Autodesk Fusion 360 part; units mm, degrees
(part 13 of 13)
  line L10724 (117.495, -110.761) -> (117.499, -110.754)
  line L10725 (117.587, -112.069) -> (117.579, -112.039)
  line L10726 (118.525, -112.429) -> (118.495, -112.435)
  line L10727 (119.85, -112.485) -> (119.85, -112.335)
  line L10728 (118.466, -112.444) -> (117.983, -112.444)
  line L10729 (117.947, -112.439) -> (117.922, -112.422)
  line L10730 (115.743, -113.759) -> (122.686, -113.759)
  line L10731 (117.956, -112.441) -> (117.954, -112.44)
  line L10732 (122.467, -112.483) -> (122.453, -112.466)
  line L10733 (123.116, -113.101) -> (123.113, -113.101)
  line L10734 (123.08, -113.084) -> (123.051, -113.068)
  line L10735 (117.506, -110.75) -> (117.513, -110.748)
  line L10736 (123.051, -113.068) -> (122.467, -112.483)
  line L10737 (117.513, -111.938) -> (117.506, -111.937)
  line L10738 (117.579, -112.039) -> (117.579, -111.938)
  line L10739 (117.513, -110.748) -> (117.873, -110.748)
  line L10740 (118.55, -112.41) -> (118.536, -112.421)
  line L10741 (122.445, -112.455) -> (122.442, -112.439)
  line L10742 (123.349, -113.096) -> (123.144, -113.104)
  line L10743 (117.881, -110.75) -> (117.887, -110.754)
  line L10744 (121.93, -112.439) -> (121.834, -112.42)
  line L10745 (118.495, -112.435) -> (118.466, -112.444)
  line L10746 (123.111, -113.101) -> (123.109, -113.1)
  line L10747 (122.453, -112.466) -> (122.45, -112.463)
  line L10748 (117.873, -110.748) -> (117.881, -110.75)
  line L10749 (120.85, -111.86) -> (120.85, -112.485)
  line L10750 (119.85, -112.335) -> (119.55, -112.335)
  line L10751 (117.887, -110.754) -> (117.892, -110.761)
  line L10752 (117.495, -111.926) -> (117.493, -111.918)
  line L10753 (117.493, -111.918) -> (117.493, -110.768)
  line L10754 (118.53, -112.425) -> (118.525, -112.429)
  line L10755 (117.602, -112.11) -> (117.598, -112.107)
  line L10756 (117.954, -112.44) -> (117.947, -112.439)
  line L10757 (117.895, -112.407) -> (117.615, -112.128)
  line L10758 (121.68, -111.86) -> (120.85, -111.86)
  line L10759 (122.686, -113.759) -> (123.349, -113.096)
  line L10760 (117.579, -111.938) -> (117.513, -111.938)
  line L10761 (117.615, -112.128) -> (117.602, -112.11)
  line L10762 (121.699, -112.284) -> (121.68, -112.189)
  line L10763 (122.449, -112.46) -> (122.445, -112.455)
  line L10764 (123.144, -113.104) -> (123.116, -113.101)
  line L10765 (117.499, -111.932) -> (117.495, -111.926)
  line L10766 (117.983, -112.444) -> (117.961, -112.441)
  line L10767 (117.598, -112.104) -> (117.594, -112.099)
  line L10768 (120.85, -112.485) -> (119.85, -112.485)
  line L10769 (117.506, -111.937) -> (117.499, -111.932)
  line L10770 (117.493, -110.768) -> (117.495, -110.761)
  line L10771 (117.598, -112.107) -> (117.598, -112.104)
  line L10772 (123.43, -112.189) -> (123.411, -112.284)
  line L10773 (125.714, -111.333) -> (125.795, -111.387)
  line L10774 (118.55, -110.985) -> (119.55, -110.985)
  line L10775 (117.829, -111.988) -> (118.035, -112.194)
  line L10776 (123.357, -111.387) -> (123.411, -111.468)
  line L10777 (120.85, -110.985) -> (120.85, -111.61)
  line L10778 (123.276, -112.42) -> (123.18, -112.439)
  line L10779 (120.85, -111.61) -> (121.68, -111.61)
  line L10780 (124.118, -112.189) -> (124.118, -111.564)
  line L10781 (123.43, -111.564) -> (123.43, -112.189)
  line L10782 (117.499, -110.754) -> (117.506, -110.75)
  line L10783 (118.414, -112.194) -> (118.55, -112.058)
  line L10784 (121.699, -111.468) -> (121.753, -111.387)
  line L10785 (124.118, -111.564) -> (124.137, -111.468)
  line L10786 (123.394, -112.83) -> (123.451, -112.719)
  line L10787 (121.68, -111.564) -> (121.699, -111.468)
  line L10788 (123.276, -111.333) -> (123.357, -111.387)
  line L10789 (117.881, -111.937) -> (117.873, -111.938)
  line L10790 (121.834, -111.333) -> (121.93, -111.314)
  line L10791 (117.892, -110.761) -> (117.893, -110.768)
  line L10792 (117.961, -112.441) -> (117.956, -112.441)
  line L10793 (117.922, -112.422) -> (117.895, -112.407)
  line L10794 (118.55, -112.058) -> (118.55, -110.985)
  line L10795 (117.873, -111.938) -> (117.829, -111.938)
  line L10796 (119.85, -110.985) -> (120.85, -110.985)
  line L10797 (119.85, -111.135) -> (119.85, -110.985)
  line L10798 (123.18, -111.314) -> (123.276, -111.333)
  line L10799 (124.192, -112.366) -> (124.137, -112.284)
  line L10800 (117.887, -111.932) -> (117.881, -111.937)
  line L10801 (119.55, -111.135) -> (119.85, -111.135)
  line L10802 (117.594, -112.099) -> (117.587, -112.069)
  line L10803 (117.829, -111.938) -> (117.829, -111.988)
  line L10804 (124.368, -112.439) -> (124.273, -112.42)
  line L10805 (117.892, -111.926) -> (117.887, -111.932)
  line L10806 (118.035, -112.194) -> (118.414, -112.194)
  line L10807 (124.273, -112.42) -> (124.192, -112.366)
  line L10808 (124.009, -112.63) -> (124.098, -112.719)
  line L10809 (117.893, -111.918) -> (117.892, -111.926)
  line L10810 (121.93, -111.314) -> (123.18, -111.314)
  line L10811 (119.55, -110.985) -> (119.55, -111.135)
  line L10812 (124.137, -111.468) -> (124.192, -111.387)
  line L10813 (123.411, -112.284) -> (123.357, -112.366)
  line L10814 (121.753, -111.387) -> (121.834, -111.333)
  line L10815 (123.411, -111.468) -> (123.43, -111.564)
  line L10816 (117.893, -110.768) -> (117.893, -111.918)
  line L10817 (121.68, -111.61) -> (121.68, -111.564)
  line L10818 (124.192, -111.387) -> (124.273, -111.333)
  line L10819 (124.273, -111.333) -> (124.368, -111.314)
  line L10820 (127.954, -111.059) -> (127.96, -111.049)
  line L10821 (123.392, -112.844) -> (123.394, -112.83)
  line L10822 (124.368, -111.314) -> (125.618, -111.314)
  line L10823 (125.618, -111.314) -> (125.714, -111.333)
  line L10824 (124.158, -113.055) -> (124.289, -113.186)
  line L10825 (128.564, -110.437) -> (128.575, -110.434)
  line L10826 (127.96, -111.049) -> (127.963, -111.038)
  line L10827 (128.538, -110.458) -> (128.564, -110.437)
  line L10828 (123.898, -112.573) -> (124.009, -112.63)
  line L10829 (125.849, -112.284) -> (125.795, -112.366)
  line L10830 (124.098, -112.719) -> (124.111, -112.745)
  line L10831 (124.771, -112.439) -> (124.159, -113.051)
  line L10832 (124.159, -113.051) -> (124.158, -113.055)
  line L10833 (128.651, -110.417) -> (136.068, -110.417)
  line L10834 (128.585, -110.428) -> (128.618, -110.424)
  line L10835 (119.55, -111.535) -> (119.55, -111.935)
  line L10836 (123.18, -112.439) -> (122.776, -112.439)
  line L10837 (123.451, -112.719) -> (123.539, -112.63)
  line L10838 (125.618, -112.439) -> (124.771, -112.439)
  line L10839 (127.273, -113.186) -> (127.943, -112.515)
  line L10840 (125.849, -111.468) -> (125.868, -111.564)
  line L10841 (124.137, -112.284) -> (124.118, -112.189)
  line L10842 (125.868, -111.564) -> (125.868, -112.189)
  line L10843 (125.868, -112.189) -> (125.849, -112.284)
  line L10844 (125.795, -111.387) -> (125.849, -111.468)
  line L10845 (123.357, -112.366) -> (123.276, -112.42)
  line L10846 (122.776, -112.439) -> (123.189, -112.852)
  line L10847 (119.85, -111.935) -> (119.85, -111.535)
  line L10848 (128.51, -110.475) -> (128.538, -110.458)
  line L10849 (136.068, -110.417) -> (136.101, -110.424)
  line L10850 (124.417, -112.439) -> (124.368, -112.439)
  line L10851 (119.85, -111.535) -> (119.55, -111.535)
  line L10852 (123.651, -112.573) -> (123.774, -112.554)
  line L10853 (123.539, -112.63) -> (123.651, -112.573)
  line L10854 (124.111, -112.745) -> (124.417, -112.439)
  line L10855 (123.774, -112.554) -> (123.898, -112.573)
  line L10856 (125.795, -112.366) -> (125.714, -112.42)
  line L10857 (128.575, -110.434) -> (128.585, -110.428)
  line L10858 (124.289, -113.186) -> (127.273, -113.186)
  line L10859 (119.55, -111.935) -> (119.85, -111.935)
  line L10860 (123.189, -112.852) -> (123.392, -112.844)
  line L10861 (128.618, -110.424) -> (128.651, -110.417)
  line L10862 (144.49, -111.398) -> (144.544, -111.479)
  line L10863 (144.544, -111.479) -> (144.563, -111.574)
  line L10864 (127.943, -111.125) -> (127.95, -111.092)
  line L10865 (125.714, -112.42) -> (125.618, -112.439)
  line L10866 (144.408, -111.343) -> (144.49, -111.398)
  line L10867 (128.002, -110.984) -> (128.51, -110.475)
  line L10868 (144.479, -113.126) -> (144.474, -113.127)
  line L10869 (145.401, -112.376) -> (145.346, -112.295)
  line L10870 (144.122, -112.449) -> (144.552, -112.88)
  line L10871 (145.465, -112.83) -> (145.485, -112.954)
  line L10872 (144.552, -112.88) -> (144.697, -112.88)
  line L10873 (145.465, -113.077) -> (145.408, -113.189)
  line L10874 (127.984, -111.012) -> (128.002, -110.984)
  line L10875 (142.832, -111.479) -> (142.886, -111.398)
  line L10876 (144.961, -113.334) -> (144.85, -113.277)
  line L10877 (145.261, -112.6) -> (145.452, -112.41)
  line L10878 (144.313, -112.449) -> (144.122, -112.449)
  line L10879 (144.85, -112.63) -> (144.961, -112.573)
  line L10880 (145.327, -111.574) -> (145.346, -111.479)
  line L10881 (144.408, -112.43) -> (144.313, -112.449)
  line L10882 (144.761, -112.719) -> (144.85, -112.63)
  line L10883 (144.961, -112.573) -> (145.085, -112.554)
  line L10884 (145.346, -112.295) -> (145.327, -112.199)
  line L10885 (146.827, -111.324) -> (146.923, -111.343)
  line L10886 (127.963, -111.038) -> (127.984, -111.012)
  line L10887 (144.49, -112.376) -> (144.408, -112.43)
  line L10888 (144.544, -112.295) -> (144.49, -112.376)
  line L10889 (145.452, -112.41) -> (145.401, -112.376)
  line L10890 (145.346, -111.479) -> (145.401, -111.398)
  line L10891 (147.077, -112.199) -> (147.058, -112.295)
  line L10892 (147.077, -111.574) -> (147.077, -112.199)
  line L10893 (144.704, -112.83) -> (144.761, -112.719)
  line L10894 (144.474, -113.127) -> (144.471, -113.125)
  line L10895 (145.327, -112.199) -> (145.327, -111.574)
  line L10896 (145.208, -112.573) -> (145.261, -112.6)
  line L10897 (144.412, -113.093) -> (143.769, -112.449)
  line L10898 (145.32, -113.277) -> (145.208, -113.334)
  line L10899 (145.766, -112.449) -> (145.438, -112.777)
  line L10900 (146.923, -111.343) -> (147.004, -111.398)
  line L10901 (144.563, -111.574) -> (144.563, -112.199)
  line L10902 (127.943, -112.515) -> (127.943, -111.125)
  line L10903 (144.563, -112.199) -> (144.544, -112.295)
  line L10904 (145.085, -112.554) -> (145.208, -112.573)
  line L10905 (145.401, -111.398) -> (145.482, -111.343)
  line L10906 (144.697, -112.88) -> (144.704, -112.83)
  line L10907 (147.058, -112.295) -> (147.004, -112.376)
  line L10908 (145.577, -111.324) -> (146.827, -111.324)
  line L10909 (147.058, -111.479) -> (147.077, -111.574)
  line L10910 (127.95, -111.092) -> (127.954, -111.059)
  line L10911 (147.004, -111.398) -> (147.058, -111.479)
  line L10912 (145.085, -113.354) -> (144.961, -113.334)
  line L10913 (144.85, -113.277) -> (144.761, -113.189)
  line L10914 (145.482, -111.343) -> (145.577, -111.324)
  line L10915 (145.408, -113.189) -> (145.32, -113.277)
  line L10916 (107.414, -117.855) -> (107.675, -118.116)
  line L10917 (107.703, -118.175) -> (107.712, -118.204)
  line L10918 (107.462, -118.256) -> (107.238, -118.032)
  line L10919 (106.661, -117.678) -> (106.681, -117.555)
  line L10920 (107.499, -122.915) -> (107.485, -122.898)
  line L10921 (107.862, -123.278) -> (107.862, -123.278)
  line L10922 (107.481, -122.892) -> (107.477, -122.887)
  line L10923 (146.78, -96.8204) -> (146.765, -96.8969)
  line L10924 (106.737, -117.913) -> (106.681, -117.802)
  line L10925 (145.98, -96.2704) -> (145.995, -96.1939)
  line L10926 (108.038, -123.102) -> (108.038, -123.102)
  line L10927 (106.737, -117.443) -> (106.826, -117.355)
  line L10928 (107.712, -118.204) -> (107.712, -122.775)
  line L10929 (108.967, -124.03) -> (141.756, -124.03)
  line L10930 (107.441, -117.802) -> (107.414, -117.855)
  line L10931 (107.471, -122.857) -> (107.462, -122.827)
  line L10932 (107.477, -122.887) -> (107.471, -122.857)
  line L10933 (146.722, -96.129) -> (146.765, -96.1939)
  line L10934 (107.238, -118.032) -> (107.185, -118.059)
  line L10935 (107.441, -117.555) -> (107.461, -117.678)
  line L10936 (108.886, -124.276) -> (108.88, -124.275)
  line L10937 (106.681, -117.555) -> (106.737, -117.443)
  line L10938 (146.18, -96.0704) -> (146.58, -96.0704)
  line L10939 (107.385, -117.443) -> (107.441, -117.555)
  line L10940 (107.461, -117.678) -> (107.441, -117.802)
  line L10941 (107.712, -122.775) -> (108.038, -123.102)
  line L10942 (107.296, -117.355) -> (107.385, -117.443)
  line L10943 (108.827, -124.244) -> (107.862, -123.278)
  line L10944 (106.681, -117.802) -> (106.661, -117.678)
  line L10945 (106.937, -117.298) -> (107.061, -117.278)
  line L10946 (145.995, -96.1939) -> (146.039, -96.129)
  line L10947 (108.889, -124.277) -> (108.886, -124.276)
  line L10948 (146.039, -96.129) -> (146.104, -96.0856)
  line L10949 (106.826, -117.355) -> (106.937, -117.298)
  line L10950 (107.697, -118.145) -> (107.703, -118.175)
  line L10951 (108.915, -124.28) -> (108.893, -124.277)
  line L10952 (107.862, -123.278) -> (107.499, -122.915)
  line L10953 (141.837, -124.272) -> (141.807, -124.28)
  line L10954 (108.88, -124.275) -> (108.854, -124.258)
sketch "Sketch2" plane through (0, 0, 0) normal (0, 0, 1) x (1, 0, 0)
  line L0 (149, -96) -> (101, -96)
  line L1 (101, -96) -> (101, -78)
  line L2 (101, -78) -> (149, -78)
  line L3 (149, -78) -> (149, -96)
  constraint horizontal L0
  constraint vertical L1
  constraint horizontal L2
  constraint vertical L3
extrude "Extrude1" add sketch "Sketch2" along normal blind 1
sketch "Sketch3" plane through (0, 0, 0) normal (0, 0, -1) x (-1, 0, 0)
  line L0 (-101, -78) -> (-149, -78)
  line L1 (-149, -78) -> (-149, -96)
  line L2 (-149, -96) -> (-101, -96)
  line L3 (-101, -96) -> (-101, -78)
  circle A0 centre (-108.7784, -82.0867) radius 0.675
  circle A1 centre (-107.4474, -84.686) radius 0.675
  circle A2 centre (-112.6298, -84.6454) radius 0.675
  circle A3 centre (-108.8729, -86.028) radius 0.675
  circle A4 centre (-107.4551, -87.3247) radius 0.675
  circle A5 centre (-111.5378, -87.2373) radius 0.675
  circle A6 centre (-112.8215, -88.5302) radius 0.675
  circle A7 centre (-111.7823, -89.8823) radius 0.675
  circle A8 centre (-108.2, -89.85) radius 0.675
  circle A9 centre (-109.8635, -92.6666) radius 0.675
  circle A10 centre (-112.05, -92.7) radius 0.675
  circle A11 centre (-114.0365, -92.6228) radius 0.675
  circle A12 centre (-117.8364, -92.898) radius 0.675
  circle A13 centre (-120.63, -92.69) radius 0.675
  circle A14 centre (-123.9456, -92.7311) radius 0.675
  circle A15 centre (-129.9244, -91.2828) radius 0.675
  circle A16 centre (-133.85, -91.1) radius 0.675
  circle A17 centre (-141.5, -92.26) radius 0.675
  circle A18 centre (-136, -83.2) radius 0.675
  circle A19 centre (-136, -86.2325) radius 0.675
  circle A20 centre (-140.7296, -81.6222) radius 0.675
  circle A21 centre (-130.6, -85.2) radius 0.675
  circle A22 centre (-129.5, -81.8) radius 0.675
  circle A23 centre (-126.6, -82.9) radius 0.675
  circle A24 centre (-124.65, -81.65) radius 0.675
  circle A25 centre (-122.1992, -81.5755) radius 0.675
  dimension "d5" = 1.35
  dimension "d6" = 1.35
  dimension "d7" = 1.35
  dimension "d8" = 1.35
  dimension "d9" = 1.35
  dimension "d10" = 1.35
  dimension "d11" = 1.35
  dimension "d12" = 1.35
  dimension "d13" = 1.35
  dimension "d14" = 1.35
  dimension "d15" = 1.35
  dimension "d16" = 1.35
  dimension "d17" = 1.35
  dimension "d18" = 1.35
  dimension "d19" = 1.35
  dimension "d20" = 1.35
  dimension "d21" = 1.35
  dimension "d22" = 1.35
  dimension "d23" = 1.35
  dimension "d24" = 1.35
  dimension "d25" = 1.35
  dimension "d26" = 1.35
  dimension "d27" = 1.35
  dimension "d28" = 1.35
  dimension "d29" = 1.35
  dimension "d30" = 1.35
  measures "d5" diameter of A0
  measures "d6" diameter of A1
  measures "d7" diameter of A3
  measures "d8" diameter of A4
  measures "d9" diameter of A2
  measures "d10" diameter of A5
  measures "d11" diameter of A6
  measures "d12" diameter of A7
  measures "d13" diameter of A8
  measures "d14" diameter of A9
  measures "d15" diameter of A10
  measures "d16" diameter of A11
  measures "d17" diameter of A12
  measures "d18" diameter of A13
  measures "d19" diameter of A14
  measures "d20" diameter of A15
  measures "d21" diameter of A21
  measures "d22" diameter of A23
  measures "d23" diameter of A24
  measures "d24" diameter of A25
  measures "d25" diameter of A22
  measures "d26" diameter of A16
  measures "d27" diameter of A19
  measures "d28" diameter of A18
  measures "d29" diameter of A20
  measures "d30" diameter of A17
sketch "Sketch4" plane through (0, 0, 0) normal (0, 0, -1) x (-1, 0, 0)
  line L0 (-101, -78) -> (-149, -78)
  line L1 (-149, -78) -> (-149, -96)
  line L2 (-149, -96) -> (-101, -96)
  line L3 (-101, -96) -> (-101, -78)
  line L4 (-101, -96) -> (-101, -78)
  line L5 (-149, -96) -> (-101, -96)
  circle A0 centre (-111.7823, -89.8823) radius 0.625
  circle A1 centre (-111.5378, -87.2373) radius 0.625
  circle A2 centre (-107.4474, -84.686) radius 0.625
  circle A3 centre (-141.5, -92.26) radius 0.625
  circle A4 centre (-107.4551, -87.3247) radius 0.625
  circle A5 centre (-108.7784, -82.0867) radius 0.625
  circle A6 centre (-112.8215, -88.5302) radius 0.625
  circle A7 centre (-109.8635, -92.6666) radius 0.625
  circle A8 centre (-122.1992, -81.5755) radius 0.625
  circle A9 centre (-112.6298, -84.6454) radius 0.625
  circle A10 centre (-108.2, -89.85) radius 0.625
  circle A11 centre (-136, -86.2325) radius 0.625
  circle A12 centre (-130.6, -85.2) radius 0.625
  circle A13 centre (-126.6, -82.9) radius 0.625
  circle A14 centre (-136, -83.2) radius 0.625
  circle A15 centre (-124.65, -81.65) radius 0.625
  circle A16 centre (-108.8729, -86.028) radius 0.625
  circle A17 centre (-133.85, -91.1) radius 0.625
  circle A18 centre (-114.0365, -92.6228) radius 0.625
  circle A19 centre (-117.8364, -92.898) radius 0.625
  circle A20 centre (-112.05, -92.7) radius 0.625
  circle A21 centre (-129.9244, -91.2828) radius 0.625
  circle A22 centre (-123.9456, -92.7311) radius 0.625
  circle A23 centre (-120.63, -92.69) radius 0.625
  circle A24 centre (-129.5, -81.8) radius 0.625
  line L6 (-149, -78) -> (-149, -96)
  circle A25 centre (-140.7296, -81.6222) radius 0.625
  line L7 (-101, -78) -> (-149, -78)
  dimension "d33" = 1.25
  dimension "d34" = 1.25
  dimension "d35" = 1.25
  dimension "d36" = 1.25
  dimension "d37" = 1.25
  dimension "d38" = 1.25
  dimension "d39" = 1.25
  dimension "d40" = 1.25
  dimension "d41" = 1.25
  dimension "d42" = 1.25
  dimension "d43" = 1.25
  dimension "d44" = 1.25
  dimension "d45" = 1.25
  dimension "d46" = 1.25
  dimension "d47" = 1.25
  dimension "d48" = 1.25
  dimension "d49" = 1.25
  dimension "d50" = 1.25
  dimension "d51" = 1.25
  dimension "d52" = 1.25
  dimension "d53" = 1.25
  dimension "d54" = 1.25
  dimension "d55" = 1.25
  dimension "d56" = 1.25
  dimension "d57" = 1.25
  dimension "d58" = 1.25
  measures "d33" diameter of A5
  measures "d34" diameter of A2
  measures "d35" diameter of A16
  measures "d36" diameter of A4
  measures "d37" diameter of A9
  measures "d38" diameter of A1
  measures "d39" diameter of A6
  measures "d40" diameter of A0
  measures "d41" diameter of A10
  measures "d42" diameter of A7
  measures "d43" diameter of A20
  measures "d44" diameter of A18
  measures "d45" diameter of A19
  measures "d46" diameter of A23
  measures "d47" diameter of A22
  measures "d48" diameter of A21
  measures "d49" diameter of A12
  measures "d50" diameter of A13
  measures "d51" diameter of A15
  measures "d52" diameter of A8
  measures "d53" diameter of A24
  measures "d54" diameter of A17
  measures "d55" diameter of A11
  measures "d56" diameter of A14
  measures "d57" diameter of A25
  measures "d58" diameter of A3
extrude "Extrude3" cut sketch "Sketch4" against normal blind 1 contours A0 | A1 | A2 | A3 | A4 | A5 | A6 | A7 | A8 | A9 | A10 | A11 | A12 | A13 | A14 | A15 | A16 | A17 | A18 | A19 | A20 | A21 | A22 | A23 | A24 | A25
sketch "Sketch5" plane through (0, 0, 0) normal (0, 0, -1) x (-1, 0, 0)
  circle A0 centre (-123.9456, -92.7311) radius 0.625
  circle A1 centre (-129.9244, -91.2828) radius 0.625
  circle A2 centre (-140.7296, -81.6222) radius 0.625
  circle A3 centre (-109.8635, -92.6666) radius 0.625
  circle A4 centre (-108.7784, -82.0867) radius 0.625
  circle A5 centre (-136, -83.2) radius 0.625
  circle A6 centre (-130.6, -85.2) radius 0.625
  circle A7 centre (-124.65, -81.65) radius 0.625
  circle A8 centre (-120.63, -92.69) radius 0.625
  circle A9 centre (-112.6298, -84.6454) radius 0.625
  circle A10 centre (-126.6, -82.9) radius 0.625
  circle A11 centre (-133.85, -91.1) radius 0.625
  circle A12 centre (-141.5, -92.26) radius 0.625
  circle A13 centre (-108.2, -89.85) radius 0.625
  circle A14 centre (-136, -86.2325) radius 0.625
  circle A15 centre (-129.5, -81.8) radius 0.625
  circle A16 centre (-122.1992, -81.5755) radius 0.625
  circle A17 centre (-117.8364, -92.898) radius 0.625
  line L0 (-101, -78) -> (-149, -78)
  line L1 (-149, -78) -> (-149, -96)
  line L2 (-149, -96) -> (-101, -96)
  line L3 (-101, -96) -> (-101, -78)
  circle A18 centre (-146, -93) radius 0.8
  circle A19 centre (-146, -80.9656) radius 0.8
  circle A20 centre (-103.4, -93) radius 0.8
  circle A21 centre (-103.4, -80.9656) radius 0.8
  circle A22 centre (-114.0365, -92.6228) radius 0.625
  circle A23 centre (-111.5378, -87.2373) radius 0.625
  circle A24 centre (-107.4474, -84.686) radius 0.625
  circle A25 centre (-112.8215, -88.5302) radius 0.625
  circle A26 centre (-112.05, -92.7) radius 0.625
  circle A27 centre (-107.4551, -87.3247) radius 0.625
  circle A28 centre (-108.8729, -86.028) radius 0.625
  circle A29 centre (-111.7823, -89.8823) radius 0.625
  dimension "d61" = 1.6
  dimension "d62" = 1.6
  dimension "d63" = 1.6
  dimension "d64" = 1.6
  dimension "d65" = 12.0344
  dimension "d66" = 3
  dimension "d67" = 3
  dimension "d120" = 42.6
  constraint vertical A20.centre A21.centre
  constraint vertical A18.centre A19.centre
  constraint horizontal A19.centre A21.centre
  constraint horizontal A18.centre A20.centre
  measures "d61" diameter of A18
  measures "d62" diameter of A19
  measures "d63" diameter of A20
  measures "d64" diameter of A21
  measures "d65" vertical distance of A18.centre A19.centre
  measures "d66" distance of L2 A18.centre
  measures "d67" distance of L1 A18.centre
  measures "d120" distance of A18.centre A20.centre
extrude "Extrude4" cut sketch "Sketch5" against normal blind 1 contours A18 | A19 | A20 | A21
extrude "Extrude5" add 1 faces at (117.7446, -87.5854, 0) along direction (0, 0, -1) blind 2.5
sketch "Sketch7" plane through (0, 0, 1) normal (0, 0, 1) x (1, 0, 0)
  line L0 (149, -78) -> (101, -78)
  line L1 (110.0613, -80.42) -> (140.0613, -80.42)
  line L2 (145.1, -83.5542) -> (145.1, -90.4251)
  line L3 (144.863, -82.792) -> (144.8869, -82.8311)
  line L4 (145.0782, -90.4018) -> (144.9206, -91.2794)
  line L5 (145.2412, -83.2117) -> (145.2415, -83.2103)
  line L6 (145.053, -83.4428) -> (145.1, -83.5542)
  line L7 (140.0273, -93.86) -> (110.0613, -93.86)
  line L8 (145.0889, -90.4512) -> (145.0782, -90.4018)
  line L9 (144.8869, -82.8311) -> (145.0095, -83.6161)
  line L10 (145.1, -90.4251) -> (145.0889, -90.4512)
  line L11 (145.0095, -83.6161) -> (145.053, -83.4428)
  arc A0 (110.0613, -80.42) -> (110.0613, -93.86) centre (110.0613, -87.14) ccw
  arc A1 (144.863, -82.792) -> (140.0613, -80.42) centre (140.0613, -86.4662) ccw
  arc A2 (140.0273, -93.86) -> (144.9206, -91.2794) centre (140.0273, -87.9303) ccw
  line L12 (101, -78) -> (149, -78)
  line L13 (149, -78) -> (149, -96)
  line L14 (149, -96) -> (101, -96)
  line L15 (101, -96) -> (101, -78)
  line L16 (149, -96) -> (149, -78)
  dimension "d73" = 6.72
  dimension "d75" = 6.0462
  dimension "d76" = 5.9297
  dimension "d77" = 5.0387
  dimension "d78" = 30
  dimension "d79" = 6.8709
  dimension "d80" = 2.42
  dimension "d81" = 3.9
  constraint horizontal L12
  constraint vertical L13
  constraint horizontal L14
  constraint vertical L15
  constraint coincident L0.end L12.start
  constraint collinear L13 L16
  constraint tangent L1 A0
  constraint tangent L1 A1
  constraint tangent L7 A0
  constraint tangent L7 A2
  constraint parallel L1 L7
  measures "d73" radius of A0
  measures "d75" radius of A1
  measures "d76" radius of A2
  measures "d77" distance of L2 A1.centre
  measures "d78" distance of L1.end L1.start
  measures "d79" distance of L2.start L2.end
  measures "d80" distance of L1 L12
  measures "d81" distance of L2 L13
extrude "Extrude6" add sketch "Sketch7" along normal blind 3
sketch "Sketch8" plane through (0, 0, -2.5) normal (0, 0, -1) x (-1, 0, 0)
  circle A0 centre (-146, -93) radius 0.8
  circle A1 centre (-146, -80.9656) radius 0.8
  circle A2 centre (-103.4, -93) radius 0.8
  circle A3 centre (-103.4, -80.9656) radius 0.8
  circle A4 centre (-123.9456, -92.7311) radius 0.625
  circle A5 centre (-129.9244, -91.2828) radius 0.625
  circle A6 centre (-140.7296, -81.6222) radius 0.625
  circle A7 centre (-109.8635, -92.6666) radius 0.625
  circle A8 centre (-108.7784, -82.0867) radius 0.625
  circle A9 centre (-136, -83.2) radius 0.625
  circle A10 centre (-130.6, -85.2) radius 0.625
  circle A11 centre (-124.65, -81.65) radius 0.625
  circle A12 centre (-120.63, -92.69) radius 0.625
  circle A13 centre (-112.6298, -84.6454) radius 0.625
  circle A14 centre (-126.6, -82.9) radius 0.625
  circle A15 centre (-133.85, -91.1) radius 0.625
  circle A16 centre (-141.5, -92.26) radius 0.625
  circle A17 centre (-108.2, -89.85) radius 0.625
  circle A18 centre (-136, -86.2325) radius 0.625
  circle A19 centre (-129.5, -81.8) radius 0.625
  circle A20 centre (-122.1992, -81.5755) radius 0.625
  circle A21 centre (-117.8364, -92.898) radius 0.625
  line L0 (-101, -78) -> (-149, -78)
  line L1 (-149, -78) -> (-149, -96)
  line L2 (-149, -96) -> (-101, -96)
  line L3 (-101, -96) -> (-101, -78)
  circle A22 centre (-103.4, -93) radius 0.8
  circle A23 centre (-146, -93) radius 0.8
  circle A24 centre (-146, -80.9656) radius 0.8
  circle A25 centre (-103.4, -80.9656) radius 0.8
  circle A26 centre (-114.0365, -92.6228) radius 0.625
  circle A27 centre (-111.5378, -87.2373) radius 0.625
  circle A28 centre (-107.4474, -84.686) radius 0.625
  circle A29 centre (-112.8215, -88.5302) radius 0.625
  circle A30 centre (-112.05, -92.7) radius 0.625
  circle A31 centre (-107.4551, -87.3247) radius 0.625
  circle A32 centre (-108.8729, -86.028) radius 0.625
  circle A33 centre (-111.7823, -89.8823) radius 0.625
  dimension "d167" = 1.6
  dimension "d168" = 1.6
  dimension "d169" = 1.6
  dimension "d170" = 1.6
  dimension "d171" = 1.6
  constraint concentric A2 A22
  constraint concentric A0 A23
  constraint concentric A1 A24
  constraint concentric A3 A25
  measures "d167" diameter of A1
  measures "d168" diameter of A24
  measures "d169" diameter of A25
  measures "d170" diameter of A22
  measures "d171" diameter of A23
extrude "Extrude7" cut sketch "Sketch8" against normal blind 20 contours A0 A23 | A1 A24 | A2 A22 | A3 A25
sketch "Sketch9" plane through (0, 0, -2.5) normal (0, 0, -1) x (-1, 0, 0)
  circle A0 centre (-146, -93) radius 0.8
  circle A1 centre (-146, -80.9656) radius 0.8
  circle A2 centre (-103.4, -93) radius 0.8
  circle A3 centre (-103.4, -80.9656) radius 0.8
  circle A4 centre (-123.9456, -92.7311) radius 0.625
  circle A5 centre (-129.9244, -91.2828) radius 0.625
  circle A6 centre (-140.7296, -81.6222) radius 0.625
  circle A7 centre (-109.8635, -92.6666) radius 0.625
  circle A8 centre (-108.7784, -82.0867) radius 0.625
  circle A9 centre (-136, -83.2) radius 0.625
  circle A10 centre (-130.6, -85.2) radius 0.625
  circle A11 centre (-124.65, -81.65) radius 0.625
  circle A12 centre (-120.63, -92.69) radius 0.625
  circle A13 centre (-112.6298, -84.6454) radius 0.625
  circle A14 centre (-126.6, -82.9) radius 0.625
  circle A15 centre (-133.85, -91.1) radius 0.625
  circle A16 centre (-141.5, -92.26) radius 0.625
  circle A17 centre (-108.2, -89.85) radius 0.625
  circle A18 centre (-136, -86.2325) radius 0.625
  circle A19 centre (-129.5, -81.8) radius 0.625
  circle A20 centre (-122.1992, -81.5755) radius 0.625
  circle A21 centre (-117.8364, -92.898) radius 0.625
  line L0 (-101, -78) -> (-149, -78)
  line L1 (-149, -78) -> (-149, -96)
  line L2 (-149, -96) -> (-101, -96)
  line L3 (-101, -96) -> (-101, -78)
  line L4 (-112.8426, -87.8084) -> (-113.7365, -88.6152)
  line L5 (-113.7365, -88.6152) -> (-112.9994, -89.4318)
  line L6 (-112.9994, -89.4318) -> (-112.1056, -88.6249)
  line L7 (-112.1056, -88.6249) -> (-112.8426, -87.8084)
  line L8 (-111.5321, -88.0445) -> (-112.3602, -87.1676)
  line L9 (-112.3602, -87.1676) -> (-112.8844, -87.6625)
  line L10 (-112.8844, -87.6625) -> (-112.0563, -88.5395)
  line L11 (-112.0563, -88.5395) -> (-111.5321, -88.0445)
  line L12 (-107.2909, -86.6561) -> (-108.3196, -87.4979)
  line L13 (-108.3196, -87.4979) -> (-108.9443, -86.7345)
  line L14 (-108.9443, -86.7345) -> (-107.9156, -85.8928)
  line L15 (-107.9156, -85.8928) -> (-107.2909, -86.6561)
  line L16 (-109.7901, -85.8311) -> (-108.8901, -86.8311)
  line L17 (-108.8901, -86.8311) -> (-113.1453, -90.6608)
  line L18 (-113.1453, -90.6608) -> (-114.0453, -89.6608)
  line L19 (-114.0453, -89.6608) -> (-109.7901, -85.8311)
  circle A22 centre (-114.0365, -92.6228) radius 0.625
  circle A23 centre (-111.5378, -87.2373) radius 0.625
  circle A24 centre (-107.4474, -84.686) radius 0.625
  circle A25 centre (-112.8215, -88.5302) radius 0.625
  circle A26 centre (-112.05, -92.7) radius 0.625
  circle A27 centre (-107.4551, -87.3247) radius 0.625
  circle A28 centre (-108.8729, -86.028) radius 0.625
  circle A29 centre (-111.7823, -89.8823) radius 0.625
  dimension "d87" = 0.55
  dimension "d88" = 0.55
  dimension "d89" = 0.55
  dimension "d90" = 0.55
  dimension "d91" = 0.55
  dimension "d92" = 0.55
  constraint perpendicular L4 L5
  constraint parallel L4 L6
  constraint parallel L5 L7
  constraint perpendicular L8 L9
  constraint parallel L8 L10
  constraint parallel L9 L11
  constraint perpendicular L12 L13
  constraint parallel L12 L14
  constraint parallel L13 L15
  constraint perpendicular L16 L17
  constraint parallel L16 L18
  constraint parallel L17 L19
  measures "d87" distance of L4 A25.centre
  measures "d88" distance of L6 A25.centre
  measures "d89" distance of L8 A23.centre
  measures "d90" distance of L10 A25.centre
  measures "d91" distance of L18 A26.centre
  measures "d92" distance of L16 A28.centre
sketch "Sketch10" plane through (0, 0, -2.5) normal (0, 0, -1) x (-1, 0, 0)
  circle A0 centre (-146, -93) radius 0.8
  circle A1 centre (-146, -80.9656) radius 0.8
  circle A2 centre (-103.4, -93) radius 0.8
  circle A3 centre (-103.4, -80.9656) radius 0.8
  circle A4 centre (-123.9456, -92.7311) radius 0.625
  circle A5 centre (-129.9244, -91.2828) radius 0.625
  circle A6 centre (-140.7296, -81.6222) radius 0.625
  circle A7 centre (-109.8635, -92.6666) radius 0.625
  circle A8 centre (-108.7784, -82.0867) radius 0.625
  circle A9 centre (-136, -83.2) radius 0.625
  circle A10 centre (-130.6, -85.2) radius 0.625
  circle A11 centre (-124.65, -81.65) radius 0.625
  circle A12 centre (-120.63, -92.69) radius 0.625
  circle A13 centre (-112.6298, -84.6454) radius 0.625
  circle A14 centre (-126.6, -82.9) radius 0.625
  circle A15 centre (-133.85, -91.1) radius 0.625
  circle A16 centre (-141.5, -92.26) radius 0.625
  circle A17 centre (-108.2, -89.85) radius 0.625
  circle A18 centre (-136, -86.2325) radius 0.625
  circle A19 centre (-129.5, -81.8) radius 0.625
  circle A20 centre (-122.1992, -81.5755) radius 0.625
  circle A21 centre (-117.8364, -92.898) radius 0.625
  line L0 (-101, -78) -> (-149, -78)
  line L1 (-149, -78) -> (-149, -96)
  line L2 (-149, -96) -> (-101, -96)
  line L3 (-101, -96) -> (-101, -78)
  line L4 (-128, -96) -> (-119, -96)
  line L5 (-119, -96) -> (-119, -99)
  line L6 (-119, -99) -> (-128, -99)
  line L7 (-128, -99) -> (-128, -96)
  line L8 (-108.5, -78) -> (-117.5, -78)
  line L9 (-117.5, -78) -> (-117.5, -75)
  line L10 (-117.5, -75) -> (-108.5, -75)
  line L11 (-108.5, -75) -> (-108.5, -78)
  circle A22 centre (-114.0365, -92.6228) radius 0.625
  circle A23 centre (-111.5378, -87.2373) radius 0.625
  circle A24 centre (-107.4474, -84.686) radius 0.625
  circle A25 centre (-112.8215, -88.5302) radius 0.625
  circle A26 centre (-112.05, -92.7) radius 0.625
  circle A27 centre (-107.4551, -87.3247) radius 0.625
  circle A28 centre (-108.8729, -86.028) radius 0.625
  circle A29 centre (-111.7823, -89.8823) radius 0.625
  dimension "d95" = 9
  dimension "d96" = 3
  dimension "d97" = 9
  dimension "d98" = 3
  dimension "d105" = 21
  dimension "d106" = 7.5
  constraint horizontal L4
  constraint vertical L5
  constraint horizontal L6
  constraint vertical L7
  constraint coincident L2 L4.start
  constraint horizontal L8
  constraint vertical L9
  constraint horizontal L10
  constraint vertical L11
  constraint coincident L0 L8.start
  measures "d95" distance of L4.start L4.end
  measures "d96" distance of L4.start L6.end
  measures "d97" distance of L8.start L8.end
  measures "d98" distance of L8.start L10.end
  measures "d105" distance of L1 L7
  measures "d106" distance of L3 L11
extrude "Extrude9" add sketch "Sketch10" against normal blind 6.5 contours L0 L8 L9 L10 L11 | L2 L4 L5 L6 L7
sketch "Sketch21" plane through (0, 0, 4) normal (0, 0, 1) x (1, 0, 0)
  circle A0 centre (103.4, -80.9656) radius 0.8
  circle A1 centre (146, -93) radius 0.8
  circle A2 centre (103.4, -93) radius 0.8
  circle A3 centre (146, -80.9656) radius 0.8
  arc A4 (110.0613, -80.42) -> (110.0613, -93.86) centre (110.0613, -87.14) ccw
  line L0 (110.0613, -80.42) -> (140.0613, -80.42)
  arc A5 (144.863, -82.792) -> (140.0613, -80.42) centre (140.0613, -86.4662) ccw
  line L1 (144.863, -82.792) -> (144.8869, -82.8311)
  line L2 (144.8869, -82.8311) -> (145.0095, -83.6161)
  line L3 (145.0095, -83.6161) -> (145.053, -83.4428)
  line L4 (145.053, -83.4428) -> (145.1, -83.5542)
  line L5 (145.1, -83.5542) -> (145.1, -90.4251)
  line L6 (145.1, -90.4251) -> (145.0889, -90.4512)
  line L7 (145.0889, -90.4512) -> (145.0782, -90.4018)
  line L8 (145.0782, -90.4018) -> (144.9206, -91.2794)
  arc A6 (140.0273, -93.86) -> (144.9206, -91.2794) centre (140.0273, -87.9303) ccw
  line L9 (140.0273, -93.86) -> (110.0613, -93.86)
  line L10 (101, -96) -> (119, -96)
  line L11 (149, -96) -> (149, -78)
  line L12 (149, -78) -> (117.5, -78)
  line L13 (101, -78) -> (101, -96)
  circle A7 centre (113, -77) radius 0.8
  circle A8 centre (123.5, -97) radius 0.8
  line L14 (119, -96) -> (119, -99)
  line L15 (119, -99) -> (128, -99)
  line L16 (128, -99) -> (128, -96)
  line L17 (128, -96) -> (149, -96)
  line L18 (117.5, -78) -> (117.5, -75)
  line L19 (117.5, -75) -> (108.5, -75)
  line L20 (108.5, -75) -> (108.5, -78)
  line L21 (108.5, -78) -> (101, -78)
  dimension "d153" = 1.6
  dimension "d154" = 1.6
  dimension "d161" = 4.5
  dimension "d162" = 9.6
  dimension "d163" = 20.1
  dimension "d164" = 3.9656
  dimension "d165" = 4
  dimension "d172" = 1.6
  measures "d153" diameter of A7
  measures "d154" diameter of A8
  measures "d161" distance of A8.centre L14
  measures "d162" horizontal distance of A0.centre A7.centre
  measures "d163" horizontal distance of A2.centre A8.centre
  measures "d164" vertical distance of A0.centre A7.centre
  measures "d165" vertical distance of A2.centre A8.centre
  measures "d172" diameter of A0
extrude "Extrude17" cut sketch "Sketch21" against normal blind 5 contours A7 | A8
sketch "Sketch22" plane through (0, 0, 1) normal (0, 0, 1) x (1, 0, 0)
  line L0 (110.0613, -93.86) -> (140.0273, -93.86)
  arc A0 (140.0273, -93.86) -> (144.9206, -91.2794) centre (140.0273, -87.9303) ccw
  line L1 (144.9206, -91.2794) -> (145.0782, -90.4018)
  line L2 (145.0782, -90.4018) -> (145.0889, -90.4512)
  line L3 (145.0889, -90.4512) -> (145.1, -90.4251)
  line L4 (145.1, -90.4251) -> (145.1, -83.5542)
  line L5 (145.1, -83.5542) -> (145.053, -83.4428)
  line L6 (145.053, -83.4428) -> (145.0095, -83.6161)
  line L7 (145.0095, -83.6161) -> (144.8869, -82.8311)
  line L8 (144.8869, -82.8311) -> (144.863, -82.792)
  arc A1 (144.863, -82.792) -> (140.0613, -80.42) centre (140.0613, -86.4662) ccw
  line L9 (140.0613, -80.42) -> (110.0613, -80.42)
  arc A2 (110.0613, -80.42) -> (110.0613, -93.86) centre (110.0613, -87.14) ccw
  circle A3 centre (123.9456, -92.7311) radius 0.625
  circle A4 centre (129.9244, -91.2828) radius 0.625
  circle A5 centre (140.7296, -81.6222) radius 0.625
  circle A6 centre (108.2, -89.85) radius 0.625
  circle A7 centre (108.7784, -82.0867) radius 0.625
  circle A8 centre (136, -83.2) radius 0.625
  circle A9 centre (130.6, -85.2) radius 0.625
  circle A10 centre (124.65, -81.65) radius 0.625
  circle A11 centre (120.63, -92.69) radius 0.625
  circle A12 centre (112.6298, -84.6454) radius 0.625
  circle A13 centre (126.6, -82.9) radius 0.625
  circle A14 centre (133.85, -91.1) radius 0.625
  circle A15 centre (141.5, -92.26) radius 0.625
  circle A16 centre (109.8635, -92.6666) radius 0.625
  circle A17 centre (136, -86.2325) radius 0.625
  circle A18 centre (129.5, -81.8) radius 0.625
  circle A19 centre (122.1992, -81.5755) radius 0.625
  circle A20 centre (114.0365, -92.6228) radius 0.625
  circle A21 centre (111.5378, -87.2373) radius 0.625
  circle A22 centre (107.4474, -84.686) radius 0.625
  circle A23 centre (112.8215, -88.5302) radius 0.625
  circle A24 centre (112.05, -92.7) radius 0.625
  circle A25 centre (107.4551, -87.3247) radius 0.625
  circle A26 centre (108.8729, -86.028) radius 0.625
  circle A27 centre (111.7823, -89.8823) radius 0.625
  circle A28 centre (117.8364, -92.898) radius 0.625
equation "d5 = d30"
equation "d6 = d30"
equation "d7 = d30"
equation "d8 = d30"
equation "d9 = d30"
equation "d10 = d30"
equation "d11 = d30"
equation "d12 = d30"
equation "d13 = d30"
equation "d14 = d30"
equation "d15 = d30"
equation "d16 = d30"
equation "d17 = d30"
equation "d18 = d30"
equation "d19 = d30"
equation "d20 = d30"
equation "d21 = d30"
equation "d22 = d30"
equation "d23 = d30"
equation "d24 = d30"
equation "d25 = d30"
equation "d26 = d30"
equation "d27 = d30"
equation "d28 = d30"
equation "d29 = d30"
equation "d33 = d58"
equation "d34 = d58"
equation "d35 = d58"
equation "d36 = d58"
equation "d37 = d58"
equation "d38 = d58"
equation "d39 = d58"
equation "d40 = d58"
equation "d41 = d58"
equation "d42 = d58"
equation "d43 = d58"
equation "d44 = d58"
equation "d45 = d58"
equation "d46 = d58"
equation "d47 = d58"
equation "d48 = d58"
equation "d49 = d58"
equation "d50 = d58"
equation "d51 = d58"
equation "d52 = d58"
equation "d53 = d58"
equation "d54 = d58"
equation "d55 = d58"
equation "d56 = d58"
equation "d57 = d58"
equation "d61 = d64"
equation "d62 = d64"
equation "d63 = d64"
equation "d87 = d92"
equation "d88 = d92"
equation "d89 = d92"
equation "d90 = d92"
equation "d91 = d92"
equation "d153 = d172"
equation "d154 = d172"
equation "d168 = d167"
equation "d169 = d167"
equation "d170 = d167"
equation "d171 = d167"
